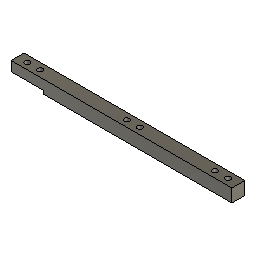
Horizontal_V10 v15 (Autodesk Fusion 360 archive; units mm, degrees)
design "MainArm_Square"
Autodesk Fusion 360 part; units mm, degrees
other "DerivedContext1"
sketch "LeftEnd" plane through (0, 0, 0) normal (1, 0, 0) x (0, 1, 0) in component "MainArm_Square"
  line L0 (-6.35, -6.35) -> (6.35, -6.35)
  line L1 (6.35, -6.35) -> (6.35, 6.35)
  line L2 (6.35, 6.35) -> (-6.35, 6.35)
  line L3 (-6.35, 6.35) -> (-6.35, -6.35)
  line L4 (-6.35, -6.35) -> (6.35, 6.35) construction
  line L5 (6.35, -6.35) -> (-6.35, 6.35) construction
  dimension "d1" = 12.7
  dimension "d2" = 12.7
  constraint horizontal L0
  constraint perpendicular L0 L1
  constraint parallel L0 L2
  constraint parallel L1 L3
  constraint coincident L4 origin
  constraint coincident L5 origin
  measures "d1" distance of L1.end L2.end
  measures "d2" distance of L0.end L1.end
sketch "Top" plane through (0, 0, 0) normal (0, 0, 1) x (1, 0, 0) in component "MainArm_Square"
  line L0 (107.95, -6.35) -> (-107.95, -6.35)
  line L1 (-107.95, -6.35) -> (-107.95, 6.35)
  line L2 (-107.95, 6.35) -> (107.95, 6.35)
  line L3 (107.95, 6.35) -> (107.95, -6.35)
  line L4 (107.95, -6.35) -> (-107.95, 6.35) construction
  line L5 (-107.95, -6.35) -> (107.95, 6.35) construction
  circle A0 centre (97.917, 0) radius 2.4892
  circle A1 centre (85.217, 0) radius 2.4892
  circle A2 centre (-98.425, 0) radius 2.4892
  circle A3 centre (-85.725, 0) radius 2.4892
  line L6 (-76.2, 6.35) -> (-76.2, -6.35)
  circle A4 centre (-1.143, 0) radius 2.4892
  circle A5 centre (11.557, 0) radius 2.4892
  dimension "d3" = 215.9
  dimension "d4" = 12.7
  dimension "d5" = 4.9784
  dimension "d6" = 4.9784
  dimension "d7" = 10.033
  dimension "d8" = 12.7
  dimension "d9" = 4.9784
  dimension "d10" = 4.9784
  dimension "d11" = 85.725
  dimension "d12" = 12.7
  dimension "d15" = 31.75
  dimension "d19" = 4.9784
  dimension "d20" = 4.9784
  dimension "d21" = 96.393
  dimension "d23" = 12.7
  constraint horizontal L0
  constraint perpendicular L0 L1
  constraint parallel L0 L2
  constraint parallel L1 L3
  constraint coincident L4 origin
  constraint coincident L5 origin
  constraint horizontal origin A0.centre
  constraint horizontal A0.centre A1.centre
  constraint horizontal origin A3.centre
  constraint horizontal A2.centre A3.centre
  constraint coincident L2 L6.start
  constraint coincident L0 L6.end
  constraint horizontal origin A4.centre
  constraint horizontal origin A5.centre
  measures "d3" distance of L1.end L2.end
  measures "d4" distance of L0.end L1.end
  measures "d5" diameter of A0
  measures "d6" diameter of A1
  measures "d7" distance of L3 A0.centre
  measures "d8" distance of A0.centre A1.centre
  measures "d9" diameter of A2
  measures "d10" diameter of A3
  measures "d11" distance of A3.centre origin
  measures "d12" distance of A2.centre A3.centre
  measures "d15" distance of L1 L6
  measures "d19" diameter of A4
  measures "d20" diameter of A5
  measures "d21" distance of L3 A5.centre
  measures "d23" distance of A4.centre A5.centre
extrude "Extrude1" add sketch "Top" along normal mid plane 12.7 in component "MainArm_Square"
extrude "Extrude2" cut sketch "Top" along normal blind 3.2614 from surface at -6.35 contours L0 L1 L2 L6 in component "MainArm_Square"
component "MainArm_Square" placed x (1, 0, 0) y (0, 1, 0) z (0, 0, 1) at (0, 0, 0)
equation "d5 = d6"
equation "d10 = d9"
equation "d19 = d6"
equation "d20 = d6"

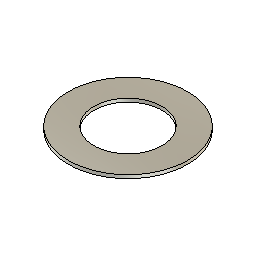
design "Washer_M4x7x0.2"
Autodesk Fusion 360 part; units mm, degrees
sketch "Sketch1" plane through (0, 0, 0) normal (0, 0, 1) x (1, 0, 0)
  circle A0 centre (0, 0) radius 2
  circle A1 centre (0, 0) radius 3.5
  dimension "d1" = 4
  dimension "d2" = 7
  constraint coincident A0.centre A1.centre
  measures "d1" diameter of A0
  measures "d2" diameter of A1
extrude "Extrude1" add sketch "Sketch1" along normal blind 0.2
